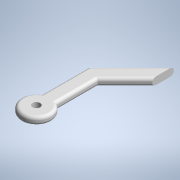
# Autodesk Inventor part: Gripper
Saved by Autodesk Inventor 2022 (Build 260153000, 153)
## iProperties
Part Number: Gripper
Material: Generic
Document SubType Name: Modeling
Designer: suhas
Appearance: Rubber - Green
Author: suhas
Autodesk Inventor part; units mm, degrees
ref_plane "YZ Plane" through (0, 0, 0) normal (1, 0, 0) x (0, 1, 0)
ref_plane "XZ Plane" through (0, 0, 0) normal (0, 1, 0) x (-1, 0, 0)
ref_plane "XY Plane" through (0, 0, 0) normal (0, 0, 1) x (1, 0, 0)
sketch "Sketch1" plane through (0, 0, 0) normal (0, 1, 0) x (-1, 0, 0)
  line L0 (5, -20) -> (5, 11.3397)
  line L1 (-5, 11.3397) -> (-5, -15.8579)
  arc A0 (5, 11.3397) -> (-5, 11.3397) centre (0, 20) ccw
  line L2 (5, -20) -> (-23.2843, -48.2843)
  line L3 (-23.2843, -34.1421) -> (-5, -15.8579)
  line L4 (5, -20) -> (45, -20) construction
  line L5 (-23.2843, -48.2843) -> (-23.2843, -34.1421)
  circle A1 centre (0, 20) radius 2.5
  point P0 (0, 0)
  dimension "d2" = 20
  dimension "d8" = 135
  dimension "d14" = 23.2843
  constraints: 12 end point, 2 centre point, 2 parallel, 2 point on circle, 1 coincident, 1 equal length, 1 horizontal, 1 vertical
  measures "d2" diameter of A0
  measures "d8" angle of L2 L4
  measures "d14" distance from line of L5 A0.centre
extrude "Extrusion1" add sketch "Sketch1" along normal blind 5
fillet "Fillet1" radius 2 10 edges at (0, 5, 30) (0, 0, 30) (5, 5, -2.2591) (-5, 5, -4.3301) (5, 0, -2.2591) (-5, 0, -4.3301) (9.1421, 0, -34.1421) (9.1421, 5, -34.1421) (14.1421, 0, -25) (14.1421, 5, -25)
body "Solid1"
